Autodesk Fusion 360 part; units mm, degrees
(part 2 of 6)
sketch "b top  projection" plane through (0, 0, 0) normal (0, 0, 1) x (1, 0, 0) in component "b top component"
  arc A0 (146.8405, 15.08) -> (148.4308, 15.08) centre (147.6356, 15.6946) ccw
  arc A1 (148.4308, 24.92) -> (146.8405, 24.92) centre (147.6356, 24.3054) ccw
  arc A2 (146.825, 24.8994) -> (146.825, 23.7113) centre (147.6356, 24.3054) ccw
  arc A3 (139.8994, 3.175) -> (138.7113, 3.175) centre (139.3054, 2.3644) ccw
  arc A4 (139.92, 1.5692) -> (139.92, 3.1595) centre (139.3054, 2.3644) ccw
  arc A5 (146.825, 36.2887) -> (146.825, 35.1006) centre (147.6356, 35.6946) ccw
  arc A6 (146.8405, 35.08) -> (148.4308, 35.08) centre (147.6356, 35.6946) ccw
  arc A7 (130.08, 3.1595) -> (130.08, 1.5692) centre (130.6946, 2.3644) ccw
  arc A8 (131.2887, 3.175) -> (130.1006, 3.175) centre (130.6946, 2.3644) ccw
  arc A9 (148.4308, 44.92) -> (146.8405, 44.92) centre (147.6356, 44.3054) ccw
  arc A10 (146.825, 44.8994) -> (146.825, 43.7113) centre (147.6356, 44.3054) ccw
  arc A11 (119.8994, 3.175) -> (118.7113, 3.175) centre (119.3054, 2.3644) ccw
  arc A12 (119.92, 1.5692) -> (119.92, 3.1595) centre (119.3054, 2.3644) ccw
  arc A13 (146.825, 56.2887) -> (146.825, 55.1006) centre (147.6356, 55.6946) ccw
  arc A14 (146.8405, 55.08) -> (148.4308, 55.08) centre (147.6356, 55.6946) ccw
  arc A15 (110.08, 3.1595) -> (110.08, 1.5692) centre (110.6946, 2.3644) ccw
  arc A16 (111.2887, 3.175) -> (110.1006, 3.175) centre (110.6946, 2.3644) ccw
  arc A17 (148.4308, 64.92) -> (146.8405, 64.92) centre (147.6356, 64.3054) ccw
  arc A18 (146.825, 64.8994) -> (146.825, 63.7113) centre (147.6356, 64.3054) ccw
  arc A19 (99.8994, 3.175) -> (98.7113, 3.175) centre (99.3054, 2.3644) ccw
  arc A20 (99.92, 1.5692) -> (99.92, 3.1595) centre (99.3054, 2.3644) ccw
  arc A21 (146.825, 76.2887) -> (146.825, 75.1006) centre (147.6356, 75.6946) ccw
  arc A22 (146.8405, 75.08) -> (148.4308, 75.08) centre (147.6356, 75.6946) ccw
  arc A23 (90.08, 3.1595) -> (90.08, 1.5692) centre (90.6946, 2.3644) ccw
  arc A24 (91.2887, 3.175) -> (90.1006, 3.175) centre (90.6946, 2.3644) ccw
  arc A25 (148.4308, 84.92) -> (146.8405, 84.92) centre (147.6356, 84.3054) ccw
  arc A26 (146.825, 84.8994) -> (146.825, 83.7113) centre (147.6356, 84.3054) ccw
  arc A27 (79.8994, 3.175) -> (78.7113, 3.175) centre (79.3054, 2.3644) ccw
  arc A28 (79.92, 1.5692) -> (79.92, 3.1595) centre (79.3054, 2.3644) ccw
  arc A29 (70.08, 3.1595) -> (70.08, 1.5692) centre (70.6946, 2.3644) ccw
  arc A30 (71.2887, 3.175) -> (70.1006, 3.175) centre (70.6946, 2.3644) ccw
  arc A31 (146.825, 96.2887) -> (146.825, 95.1006) centre (147.6356, 95.6946) ccw
  arc A32 (146.8405, 95.08) -> (148.4308, 95.08) centre (147.6356, 95.6946) ccw
  arc A33 (148.4308, 104.92) -> (146.8405, 104.92) centre (147.6356, 104.3054) ccw
  arc A34 (146.825, 104.8994) -> (146.825, 103.7113) centre (147.6356, 104.3054) ccw
  arc A35 (59.8994, 3.175) -> (58.7113, 3.175) centre (59.3054, 2.3644) ccw
  arc A36 (59.92, 1.5692) -> (59.92, 3.1595) centre (59.3054, 2.3644) ccw
  arc A37 (50.08, 3.1595) -> (50.08, 1.5692) centre (50.6946, 2.3644) ccw
  arc A38 (51.2887, 3.175) -> (50.1006, 3.175) centre (50.6946, 2.3644) ccw
  arc A39 (138.7113, 116.825) -> (139.8994, 116.825) centre (139.3054, 117.6356) ccw
  arc A40 (139.92, 116.8405) -> (139.92, 118.4308) centre (139.3054, 117.6356) ccw
  arc A41 (39.8994, 3.175) -> (38.7113, 3.175) centre (39.3054, 2.3644) ccw
  arc A42 (39.92, 1.5692) -> (39.92, 3.1595) centre (39.3054, 2.3644) ccw
  arc A43 (130.08, 118.4308) -> (130.08, 116.8405) centre (130.6946, 117.6356) ccw
  arc A44 (130.1006, 116.825) -> (131.2887, 116.825) centre (130.6946, 117.6356) ccw
  arc A45 (30.08, 3.1595) -> (30.08, 1.5692) centre (30.6946, 2.3644) ccw
  arc A46 (31.2887, 3.175) -> (30.1006, 3.175) centre (30.6946, 2.3644) ccw
  arc A47 (118.7113, 116.825) -> (119.8994, 116.825) centre (119.3054, 117.6356) ccw
  arc A48 (119.92, 116.8405) -> (119.92, 118.4308) centre (119.3054, 117.6356) ccw
  arc A49 (19.8994, 3.175) -> (18.7113, 3.175) centre (19.3054, 2.3644) ccw
  arc A50 (19.92, 1.5692) -> (19.92, 3.1595) centre (19.3054, 2.3644) ccw
  arc A51 (110.08, 118.4308) -> (110.08, 116.8405) centre (110.6946, 117.6356) ccw
  arc A52 (110.1006, 116.825) -> (111.2887, 116.825) centre (110.6946, 117.6356) ccw
  arc A53 (10.08, 3.1595) -> (10.08, 1.5692) centre (10.6946, 2.3644) ccw
  arc A54 (11.2887, 3.175) -> (10.1006, 3.175) centre (10.6946, 2.3644) ccw
  arc A55 (98.7113, 116.825) -> (99.8994, 116.825) centre (99.3054, 117.6356) ccw
  arc A56 (99.92, 116.8405) -> (99.92, 118.4308) centre (99.3054, 117.6356) ccw
  arc A57 (90.08, 118.4308) -> (90.08, 116.8405) centre (90.6946, 117.6356) ccw
  arc A58 (90.1006, 116.825) -> (91.2887, 116.825) centre (90.6946, 117.6356) ccw
  arc A59 (3.175, 15.1006) -> (3.175, 16.2887) centre (2.3644, 15.6946) ccw
  arc A60 (1.5692, 15.08) -> (3.1595, 15.08) centre (2.3644, 15.6946) ccw
  arc A61 (3.1595, 24.92) -> (1.5692, 24.92) centre (2.3644, 24.3054) ccw
  arc A62 (3.175, 23.7113) -> (3.175, 24.8994) centre (2.3644, 24.3054) ccw
  arc A63 (78.7113, 116.825) -> (79.8994, 116.825) centre (79.3054, 117.6356) ccw
  arc A64 (79.92, 116.8405) -> (79.92, 118.4308) centre (79.3054, 117.6356) ccw
  arc A65 (3.175, 35.1006) -> (3.175, 36.2887) centre (2.3644, 35.6946) ccw
  arc A66 (1.5692, 35.08) -> (3.1595, 35.08) centre (2.3644, 35.6946) ccw
  arc A67 (70.08, 118.4308) -> (70.08, 116.8405) centre (70.6946, 117.6356) ccw
  arc A68 (70.1006, 116.825) -> (71.2887, 116.825) centre (70.6946, 117.6356) ccw
  arc A69 (3.1595, 44.92) -> (1.5692, 44.92) centre (2.3644, 44.3054) ccw
  arc A70 (3.175, 43.7113) -> (3.175, 44.8994) centre (2.3644, 44.3054) ccw
  arc A71 (58.7113, 116.825) -> (59.8994, 116.825) centre (59.3054, 117.6356) ccw
  arc A72 (59.92, 116.8405) -> (59.92, 118.4308) centre (59.3054, 117.6356) ccw
  arc A73 (3.175, 55.1006) -> (3.175, 56.2887) centre (2.3644, 55.6946) ccw
  arc A74 (1.5692, 55.08) -> (3.1595, 55.08) centre (2.3644, 55.6946) ccw
  arc A75 (50.08, 118.4308) -> (50.08, 116.8405) centre (50.6946, 117.6356) ccw
  arc A76 (50.1006, 116.825) -> (51.2887, 116.825) centre (50.6946, 117.6356) ccw
  arc A77 (3.1595, 64.92) -> (1.5692, 64.92) centre (2.3644, 64.3054) ccw
  arc A78 (3.175, 63.7113) -> (3.175, 64.8994) centre (2.3644, 64.3054) ccw
  arc A79 (38.7113, 116.825) -> (39.8994, 116.825) centre (39.3054, 117.6356) ccw
  arc A80 (39.92, 116.8405) -> (39.92, 118.4308) centre (39.3054, 117.6356) ccw
  arc A81 (3.175, 75.1006) -> (3.175, 76.2887) centre (2.3644, 75.6946) ccw
  arc A82 (1.5692, 75.08) -> (3.1595, 75.08) centre (2.3644, 75.6946) ccw
  arc A83 (30.08, 118.4308) -> (30.08, 116.8405) centre (30.6946, 117.6356) ccw
  arc A84 (30.1006, 116.825) -> (31.2887, 116.825) centre (30.6946, 117.6356) ccw
  arc A85 (3.1595, 84.92) -> (1.5692, 84.92) centre (2.3644, 84.3054) ccw
  arc A86 (3.175, 83.7113) -> (3.175, 84.8994) centre (2.3644, 84.3054) ccw
  arc A87 (18.7113, 116.825) -> (19.8994, 116.825) centre (19.3054, 117.6356) ccw
  arc A88 (19.92, 116.8405) -> (19.92, 118.4308) centre (19.3054, 117.6356) ccw
  arc A89 (3.175, 95.1006) -> (3.175, 96.2887) centre (2.3644, 95.6946) ccw
  arc A90 (1.5692, 95.08) -> (3.1595, 95.08) centre (2.3644, 95.6946) ccw
  arc A91 (10.08, 118.4308) -> (10.08, 116.8405) centre (10.6946, 117.6356) ccw
  arc A92 (10.1006, 116.825) -> (11.2887, 116.825) centre (10.6946, 117.6356) ccw
  arc A93 (3.1595, 104.92) -> (1.5692, 104.92) centre (2.3644, 104.3054) ccw
  arc A94 (3.175, 103.7113) -> (3.175, 104.8994) centre (2.3644, 104.3054) ccw
  arc A95 (146.825, 16.2887) -> (146.825, 15.1006) centre (147.6356, 15.6946) ccw
  line L0 (150, 15.08) -> (148.4308, 15.08)
  line L1 (146.825, 24.8994) -> (146.825, 24.92)
  line L2 (146.825, 16.2887) -> (146.825, 23.7113)
  line L3 (146.825, 15.08) -> (146.825, 15.1006)
  line L4 (148.4308, 24.92) -> (150, 24.92)
  line L5 (139.92, 3.175) -> (139.92, 3.1595)
  line L6 (146.8405, 35.08) -> (146.825, 35.08)
  line L7 (130.08, 3.175) -> (130.1006, 3.175)
  line L8 (131.2887, 3.175) -> (138.7113, 3.175)
  line L9 (130.08, 0) -> (130.08, 1.5692)
  line L10 (146.825, 44.8994) -> (146.825, 44.92)
  line L11 (146.825, 36.2887) -> (146.825, 43.7113)
  line L12 (148.4308, 44.92) -> (150, 44.92)
  line L13 (119.92, 3.175) -> (119.92, 3.1595)
  line L14 (146.8405, 55.08) -> (146.825, 55.08)
  line L15 (110.08, 3.175) -> (110.1006, 3.175)
  line L16 (111.2887, 3.175) -> (118.7113, 3.175)
  line L17 (110.08, 0) -> (110.08, 1.5692)
  line L18 (146.825, 64.8994) -> (146.825, 64.92)
  line L19 (146.825, 56.2887) -> (146.825, 63.7113)
  line L20 (99.92, 3.175) -> (99.92, 3.1595)
  line L21 (148.4308, 64.92) -> (150, 64.92)
  line L22 (146.8405, 75.08) -> (146.825, 75.08)
  line L23 (90.08, 3.175) -> (90.1006, 3.175)
  line L24 (91.2887, 3.175) -> (98.7113, 3.175)
  line L25 (90.08, 0) -> (90.08, 1.5692)
  line L26 (146.825, 84.8994) -> (146.825, 84.92)
  line L27 (146.825, 76.2887) -> (146.825, 83.7113)
  line L28 (79.92, 3.175) -> (79.92, 3.1595)
  line L29 (148.4308, 84.92) -> (150, 84.92)
  line L30 (70.08, 3.175) -> (70.1006, 3.175)
  line L31 (71.2887, 3.175) -> (78.7113, 3.175)
  line L32 (146.8405, 95.08) -> (146.825, 95.08)
  line L33 (70.08, 0) -> (70.08, 1.5692)
  line L34 (146.825, 104.8994) -> (146.825, 104.92)
  line L35 (146.825, 96.2887) -> (146.825, 103.7113)
  line L36 (59.92, 3.175) -> (59.92, 3.1595)
  line L37 (148.4308, 104.92) -> (150, 104.92)
  line L38 (50.08, 3.175) -> (50.1006, 3.175)
  line L39 (51.2887, 3.175) -> (58.7113, 3.175)
  line L40 (139.92, 116.825) -> (139.92, 116.8405)
  line L41 (50.08, 0) -> (50.08, 1.5692)
  line L42 (130.08, 116.825) -> (130.1006, 116.825)
  line L43 (131.2887, 116.825) -> (138.7113, 116.825)
  line L44 (39.92, 3.175) -> (39.92, 3.1595)
  line L45 (130.08, 120) -> (130.08, 118.4308)
  line L46 (30.08, 3.175) -> (30.1006, 3.175)
  line L47 (31.2887, 3.175) -> (38.7113, 3.175)
  line L48 (119.92, 116.825) -> (119.92, 116.8405)
  line L49 (30.08, 0) -> (30.08, 1.5692)
  line L50 (110.08, 116.825) -> (110.1006, 116.825)
  line L51 (111.2887, 116.825) -> (118.7113, 116.825)
  line L52 (19.92, 3.175) -> (19.92, 3.1595)
  line L53 (110.08, 120) -> (110.08, 118.4308)
  line L54 (10.08, 3.175) -> (10.1006, 3.175)
  line L55 (11.2887, 3.175) -> (18.7113, 3.175)
  line L56 (99.92, 116.825) -> (99.92, 116.8405)
  line L57 (10.08, 0) -> (10.08, 1.5692)
  line L58 (90.08, 116.825) -> (90.1006, 116.825)
  line L59 (91.2887, 116.825) -> (98.7113, 116.825)
  line L60 (3.1595, 15.08) -> (3.175, 15.08)
  line L61 (90.08, 120) -> (90.08, 118.4308)
  line L62 (3.175, 24.8994) -> (3.175, 24.92)
  line L63 (3.175, 16.2887) -> (3.175, 23.7113)
  line L64 (79.92, 116.825) -> (79.92, 116.8405)
  line L65 (1.5692, 24.92) -> (0, 24.92)
  line L66 (70.08, 116.825) -> (70.1006, 116.825)
  line L67 (71.2887, 116.825) -> (78.7113, 116.825)
  line L68 (3.1595, 35.08) -> (3.175, 35.08)
  line L69 (70.08, 120) -> (70.08, 118.4308)
  line L70 (3.175, 44.8994) -> (3.175, 44.92)
  line L71 (3.175, 36.2887) -> (3.175, 43.7113)
  line L72 (59.92, 116.825) -> (59.92, 116.8405)
  line L73 (1.5692, 44.92) -> (0, 44.92)
  line L74 (3.1595, 55.08) -> (3.175, 55.08)
  line L75 (50.08, 116.825) -> (50.1006, 116.825)
  line L76 (51.2887, 116.825) -> (58.7113, 116.825)
  line L77 (50.08, 120) -> (50.08, 118.4308)
  line L78 (3.175, 64.8994) -> (3.175, 64.92)
  line L79 (3.175, 56.2887) -> (3.175, 63.7113)
  line L80 (1.5692, 64.92) -> (0, 64.92)
  line L81 (39.92, 116.825) -> (39.92, 116.8405)
  line L82 (3.1595, 75.08) -> (3.175, 75.08)
  line L83 (30.08, 116.825) -> (30.1006, 116.825)
  line L84 (31.2887, 116.825) -> (38.7113, 116.825)
  line L85 (3.175, 84.8994) -> (3.175, 84.92)
  line L86 (3.175, 76.2887) -> (3.175, 83.7113)
  line L87 (30.08, 120) -> (30.08, 118.4308)
  line L88 (1.5692, 84.92) -> (0, 84.92)
  line L89 (19.92, 116.825) -> (19.92, 116.8405)
  line L90 (3.1595, 95.08) -> (3.175, 95.08)
  line L91 (10.08, 116.825) -> (10.1006, 116.825)
  line L92 (11.2887, 116.825) -> (18.7113, 116.825)
  line L93 (3.175, 104.8994) -> (3.175, 104.92)
  line L94 (3.175, 96.2887) -> (3.175, 103.7113)
  line L95 (10.08, 120) -> (10.08, 118.4308)
  line L96 (1.5692, 104.92) -> (0, 104.92)
  line L97 (0, 0) -> (0, 15.08)
  line L98 (0, 15.08) -> (1.5692, 15.08)
  line L99 (3.175, 15.08) -> (3.175, 15.1006)
  line L100 (3.175, 24.92) -> (3.1595, 24.92)
  line L101 (0, 24.92) -> (0, 35.08)
  line L102 (0, 35.08) -> (1.5692, 35.08)
  line L103 (3.175, 35.08) -> (3.175, 35.1006)
  line L104 (3.175, 44.92) -> (3.1595, 44.92)
  line L105 (0, 44.92) -> (0, 55.08)
  line L106 (0, 55.08) -> (1.5692, 55.08)
  line L107 (3.175, 55.08) -> (3.175, 55.1006)
  line L108 (3.175, 64.92) -> (3.1595, 64.92)
  line L109 (0, 64.92) -> (0, 75.08)
  line L110 (0, 75.08) -> (1.5692, 75.08)
  line L111 (3.175, 75.08) -> (3.175, 75.1006)
  line L112 (3.175, 84.92) -> (3.1595, 84.92)
  line L113 (0, 84.92) -> (0, 95.08)
  line L114 (0, 95.08) -> (1.5692, 95.08)
  line L115 (3.175, 95.08) -> (3.175, 95.1006)
  line L116 (3.175, 104.92) -> (3.1595, 104.92)
  line L117 (0, 104.92) -> (0, 120)
  line L118 (0, 120) -> (10.08, 120)
  line L119 (10.08, 116.8405) -> (10.08, 116.825)
  line L120 (19.8994, 116.825) -> (19.92, 116.825)
  line L121 (19.92, 118.4308) -> (19.92, 120)
  line L122 (19.92, 120) -> (30.08, 120)
  line L123 (30.08, 116.8405) -> (30.08, 116.825)
  line L124 (39.8994, 116.825) -> (39.92, 116.825)
  line L125 (39.92, 118.4308) -> (39.92, 120)
  line L126 (39.92, 120) -> (50.08, 120)
  line L127 (50.08, 116.8405) -> (50.08, 116.825)
  line L128 (59.8994, 116.825) -> (59.92, 116.825)
  line L129 (59.92, 118.4308) -> (59.92, 120)
  line L130 (59.92, 120) -> (70.08, 120)
  line L131 (70.08, 116.8405) -> (70.08, 116.825)
  line L132 (79.8994, 116.825) -> (79.92, 116.825)
  line L133 (79.92, 118.4308) -> (79.92, 120)
  line L134 (79.92, 120) -> (90.08, 120)
  line L135 (90.08, 116.8405) -> (90.08, 116.825)
  line L136 (99.8994, 116.825) -> (99.92, 116.825)
  line L137 (99.92, 118.4308) -> (99.92, 120)
  line L138 (99.92, 120) -> (110.08, 120)
  line L139 (110.08, 116.8405) -> (110.08, 116.825)
  line L140 (119.8994, 116.825) -> (119.92, 116.825)
  line L141 (119.92, 118.4308) -> (119.92, 120)
  line L142 (119.92, 120) -> (130.08, 120)
  line L143 (130.08, 116.8405) -> (130.08, 116.825)
  line L144 (139.8994, 116.825) -> (139.92, 116.825)
  line L145 (139.92, 118.4308) -> (139.92, 120)
  line L146 (139.92, 120) -> (150, 120)
  line L147 (150, 104.92) -> (150, 120)
  line L148 (146.825, 104.92) -> (146.8405, 104.92)
  line L149 (146.825, 95.08) -> (146.825, 95.1006)
  line L150 (150, 95.08) -> (148.4308, 95.08)
  line L151 (150, 84.92) -> (150, 95.08)
  line L152 (146.825, 84.92) -> (146.8405, 84.92)
  line L153 (146.825, 75.08) -> (146.825, 75.1006)
  line L154 (150, 75.08) -> (148.4308, 75.08)
  line L155 (150, 64.92) -> (150, 75.08)
  line L156 (146.825, 64.92) -> (146.8405, 64.92)
  line L157 (146.825, 55.08) -> (146.825, 55.1006)
  line L158 (150, 55.08) -> (148.4308, 55.08)
  line L159 (150, 44.92) -> (150, 55.08)
  line L160 (146.825, 44.92) -> (146.8405, 44.92)
  line L161 (146.825, 35.08) -> (146.825, 35.1006)
  line L162 (150, 35.08) -> (148.4308, 35.08)
  line L163 (150, 24.92) -> (150, 35.08)
  line L164 (146.825, 24.92) -> (146.8405, 24.92)
  line L165 (146.8405, 15.08) -> (146.825, 15.08)
  line L166 (150, 0) -> (150, 15.08)
  line L167 (139.92, 0) -> (150, 0)
  line L168 (139.92, 1.5692) -> (139.92, 0)
  line L169 (139.8994, 3.175) -> (139.92, 3.175)
  line L170 (130.08, 3.1595) -> (130.08, 3.175)
  line L171 (119.92, 0) -> (130.08, 0)
  line L172 (119.92, 1.5692) -> (119.92, 0)
  line L173 (119.8994, 3.175) -> (119.92, 3.175)
  line L174 (110.08, 3.1595) -> (110.08, 3.175)
  line L175 (99.92, 0) -> (110.08, 0)
  line L176 (99.92, 1.5692) -> (99.92, 0)
  line L177 (99.8994, 3.175) -> (99.92, 3.175)
  line L178 (90.08, 3.1595) -> (90.08, 3.175)
  line L179 (79.92, 0) -> (90.08, 0)
  line L180 (79.92, 1.5692) -> (79.92, 0)
  line L181 (79.8994, 3.175) -> (79.92, 3.175)
  line L182 (70.08, 3.1595) -> (70.08, 3.175)
  line L183 (59.92, 0) -> (70.08, 0)
  line L184 (59.92, 1.5692) -> (59.92, 0)
  line L185 (59.8994, 3.175) -> (59.92, 3.175)
  line L186 (50.08, 3.1595) -> (50.08, 3.175)
  line L187 (39.92, 0) -> (50.08, 0)
  line L188 (39.92, 1.5692) -> (39.92, 0)
  line L189 (39.8994, 3.175) -> (39.92, 3.175)
  line L190 (30.08, 3.1595) -> (30.08, 3.175)
  line L191 (19.92, 0) -> (30.08, 0)
  line L192 (19.92, 1.5692) -> (19.92, 0)
  line L193 (19.8994, 3.175) -> (19.92, 3.175)
  line L194 (10.08, 3.1595) -> (10.08, 3.175)
  line L195 (0, 0) -> (10.08, 0)
sketch "b bottom lines" plane through (0, 0, 0) normal (0, 0, 1) x (1, 0, 0) in component "b bottom component"
  line L0 (152.01, 0) -> (162.09, 0)
  line L1 (162.09, 0) -> (162.09, 3.175)
  line L2 (162.09, 3.175) -> (171.93, 3.175)
  line L3 (171.93, 3.175) -> (171.93, 0)
  line L4 (171.93, 0) -> (182.09, 0)
  line L5 (182.09, 0) -> (182.09, 3.175)
  line L6 (182.09, 3.175) -> (191.93, 3.175)
  line L7 (191.93, 3.175) -> (191.93, 0)
  line L8 (191.93, 0) -> (202.09, 0)
  line L9 (202.09, 0) -> (202.09, 3.175)
  line L10 (202.09, 3.175) -> (211.93, 3.175)
  line L11 (211.93, 3.175) -> (211.93, 0)
  line L12 (211.93, 0) -> (222.09, 0)
  line L13 (222.09, 0) -> (222.09, 3.175)
  line L14 (222.09, 3.175) -> (231.93, 3.175)
  line L15 (231.93, 3.175) -> (231.93, 0)
  line L16 (231.93, 0) -> (242.09, 0)
  line L17 (242.09, 0) -> (242.09, 3.175)
  line L18 (242.09, 3.175) -> (251.93, 3.175)
  line L19 (251.93, 3.175) -> (251.93, 0)
  line L20 (251.93, 0) -> (262.09, 0)
  line L21 (262.09, 0) -> (262.09, 3.175)
  line L22 (262.09, 3.175) -> (271.93, 3.175)
  line L23 (271.93, 3.175) -> (271.93, 0)
  line L24 (271.93, 0) -> (282.09, 0)
  line L25 (282.09, 0) -> (282.09, 3.175)
  line L26 (282.09, 3.175) -> (291.93, 3.175)
  line L27 (291.93, 3.175) -> (291.93, 0)
  line L28 (291.93, 0) -> (302.01, 0)
  line L29 (302.01, 0) -> (302.01, 15.08)
  line L30 (302.01, 15.08) -> (298.835, 15.08)
  line L31 (298.835, 15.08) -> (298.835, 24.92)
  line L32 (298.835, 24.92) -> (302.01, 24.92)
  line L33 (302.01, 24.92) -> (302.01, 35.08)
  line L34 (302.01, 35.08) -> (298.835, 35.08)
  line L35 (298.835, 35.08) -> (298.835, 44.92)
  line L36 (298.835, 44.92) -> (302.01, 44.92)
  line L37 (302.01, 44.92) -> (302.01, 55.08)
  line L38 (302.01, 55.08) -> (298.835, 55.08)
  line L39 (298.835, 55.08) -> (298.835, 64.92)
  line L40 (298.835, 64.92) -> (302.01, 64.92)
  line L41 (302.01, 64.92) -> (302.01, 75.08)
  line L42 (302.01, 75.08) -> (298.835, 75.08)
  line L43 (298.835, 75.08) -> (298.835, 84.92)
  line L44 (298.835, 84.92) -> (302.01, 84.92)
  line L45 (302.01, 84.92) -> (302.01, 95.08)
  line L46 (302.01, 95.08) -> (298.835, 95.08)
  line L47 (298.835, 95.08) -> (298.835, 104.92)
  line L48 (298.835, 104.92) -> (302.01, 104.92)
  line L49 (302.01, 104.92) -> (302.01, 120)
  line L50 (152.01, 120) -> (162.09, 120)
  line L51 (162.09, 120) -> (162.09, 116.825)
  line L52 (162.09, 116.825) -> (171.93, 116.825)
  line L53 (171.93, 116.825) -> (171.93, 120)
  line L54 (171.93, 120) -> (182.09, 120)
  line L55 (182.09, 120) -> (182.09, 116.825)
  line L56 (182.09, 116.825) -> (191.93, 116.825)
  line L57 (191.93, 116.825) -> (191.93, 120)
  line L58 (191.93, 120) -> (202.09, 120)
  line L59 (202.09, 120) -> (202.09, 116.825)
  line L60 (202.09, 116.825) -> (211.93, 116.825)
  line L61 (211.93, 116.825) -> (211.93, 120)
  line L62 (211.93, 120) -> (222.09, 120)
  line L63 (222.09, 120) -> (222.09, 116.825)
  line L64 (222.09, 116.825) -> (231.93, 116.825)
  line L65 (231.93, 116.825) -> (231.93, 120)
  line L66 (231.93, 120) -> (242.09, 120)
  line L67 (242.09, 120) -> (242.09, 116.825)
  line L68 (242.09, 116.825) -> (251.93, 116.825)
  line L69 (251.93, 116.825) -> (251.93, 120)
  line L70 (251.93, 120) -> (262.09, 120)
  line L71 (262.09, 120) -> (262.09, 116.825)
  line L72 (262.09, 116.825) -> (271.93, 116.825)
  line L73 (271.93, 116.825) -> (271.93, 120)
  line L74 (271.93, 120) -> (282.09, 120)
  line L75 (282.09, 120) -> (282.09, 116.825)
  line L76 (282.09, 116.825) -> (291.93, 116.825)
  line L77 (291.93, 116.825) -> (291.93, 120)
  line L78 (291.93, 120) -> (302.01, 120)
  line L79 (152.01, 0) -> (152.01, 15.08)
  line L80 (152.01, 15.08) -> (155.185, 15.08)
  line L81 (155.185, 15.08) -> (155.185, 24.92)
  line L82 (155.185, 24.92) -> (152.01, 24.92)
  line L83 (152.01, 24.92) -> (152.01, 35.08)
  line L84 (152.01, 35.08) -> (155.185, 35.08)
  line L85 (155.185, 35.08) -> (155.185, 44.92)
  line L86 (155.185, 44.92) -> (152.01, 44.92)
  line L87 (152.01, 44.92) -> (152.01, 55.08)
  line L88 (152.01, 55.08) -> (155.185, 55.08)
  line L89 (155.185, 55.08) -> (155.185, 64.92)
  line L90 (155.185, 64.92) -> (152.01, 64.92)
  line L91 (152.01, 64.92) -> (152.01, 75.08)
  line L92 (152.01, 75.08) -> (155.185, 75.08)
  line L93 (155.185, 75.08) -> (155.185, 84.92)
  line L94 (155.185, 84.92) -> (152.01, 84.92)
  line L95 (152.01, 84.92) -> (152.01, 95.08)
  line L96 (152.01, 95.08) -> (155.185, 95.08)
  line L97 (155.185, 95.08) -> (155.185, 104.92)
  line L98 (155.185, 104.92) -> (152.01, 104.92)
  line L99 (152.01, 104.92) -> (152.01, 120)
  dimension "d5342" = 10.08
  dimension "d5343" = 3.175
  dimension "d5344" = 9.84
  dimension "d5345" = 3.175
  dimension "d5346" = 10.16
  dimension "d5347" = 3.175
  dimension "d5348" = 9.84
  dimension "d5349" = 3.175
  dimension "d5350" = 10.16
  dimension "d5351" = 3.175
  dimension "d5352" = 9.84
  dimension "d5353" = 3.175
  dimension "d5354" = 10.16
  dimension "d5355" = 3.175
  dimension "d5356" = 9.84
  dimension "d5357" = 3.175
  dimension "d5358" = 10.16
  dimension "d5359" = 3.175
  dimension "d5360" = 9.84
  dimension "d5361" = 3.175
  dimension "d5362" = 10.16
  dimension "d5363" = 3.175
  dimension "d5364" = 9.84
  dimension "d5365" = 3.175
  dimension "d5366" = 10.16
  dimension "d5367" = 3.175
  dimension "d5368" = 9.84
  dimension "d5369" = 3.175
  dimension "d5370" = 10.08
  dimension "d5385" = 15.08
  dimension "d5386" = 3.175
  dimension "d5387" = 9.84
  dimension "d5388" = 3.175
  dimension "d5389" = 10.16
  dimension "d5390" = 3.175
  dimension "d5391" = 9.84
  dimension "d5392" = 3.175
  dimension "d5393" = 10.16
  dimension "d5394" = 3.175
  dimension "d5395" = 9.84
  dimension "d5396" = 3.175
  dimension "d5397" = 10.16
  dimension "d5398" = 3.175
  dimension "d5399" = 9.84
  dimension "d5400" = 3.175
  dimension "d5401" = 10.16
  dimension "d5402" = 3.175
  dimension "d5403" = 9.84
  dimension "d5404" = 3.175
  dimension "d5405" = 15.08
  dimension "d5416" = 10.08
  dimension "d5417" = 3.175
  dimension "d5418" = 9.84
  dimension "d5419" = 3.175
  dimension "d5420" = 10.16
  dimension "d5421" = 3.175
  dimension "d5422" = 9.84
  dimension "d5423" = 3.175
  dimension "d5424" = 10.16
  dimension "d5425" = 3.175
  dimension "d5426" = 9.84
  dimension "d5427" = 3.175
  dimension "d5428" = 10.16
  dimension "d5429" = 3.175
  dimension "d5430" = 9.84
  dimension "d5431" = 3.175
  dimension "d5432" = 10.16
  dimension "d5433" = 3.175
  dimension "d5434" = 9.84
  dimension "d5435" = 3.175
  dimension "d5436" = 10.16
  dimension "d5437" = 3.175
  dimension "d5438" = 9.84
  dimension "d5439" = 3.175
  dimension "d5440" = 10.16
  dimension "d5441" = 3.175
  dimension "d5442" = 9.84
  dimension "d5443" = 3.175
  dimension "d5444" = 10.08
  dimension "d5459" = 15.08
  dimension "d5460" = 3.175
  dimension "d5461" = 9.84
  dimension "d5462" = 3.175
  dimension "d5463" = 10.16
  dimension "d5464" = 3.175
  dimension "d5465" = 9.84
  dimension "d5466" = 3.175
  dimension "d5467" = 10.16
  dimension "d5468" = 3.175
  dimension "d5469" = 9.84
  dimension "d5470" = 3.175
  dimension "d5471" = 10.16
  dimension "d5472" = 3.175
  dimension "d5473" = 9.84
  dimension "d5474" = 3.175
  dimension "d5475" = 10.16
  dimension "d5476" = 3.175
  dimension "d5477" = 9.84
  dimension "d5478" = 3.175
  dimension "d5479" = 15.08
  constraint horizontal L0
  constraint vertical L1
  constraint horizontal L2
  constraint vertical L3
  constraint horizontal L4
  constraint vertical L5
  constraint horizontal L6
  constraint vertical L7
  constraint horizontal L8
  constraint vertical L9
  constraint horizontal L10
  constraint vertical L11
  constraint horizontal L12
  constraint vertical L13
  constraint horizontal L14
  constraint vertical L15
  constraint horizontal L16
  constraint vertical L17
  constraint horizontal L18
  constraint vertical L19
  constraint horizontal L20
  constraint vertical L21
  constraint horizontal L22
  constraint vertical L23
  constraint horizontal L24
  constraint vertical L25
  constraint horizontal L26
  constraint vertical L27
  constraint horizontal L28
  constraint vertical L29
  constraint horizontal L30
  constraint vertical L31
  constraint horizontal L32
  constraint vertical L33
  constraint horizontal L34
  constraint vertical L35
  constraint horizontal L36
  constraint vertical L37
  constraint horizontal L38
  constraint vertical L39
  constraint horizontal L40
  constraint vertical L41
  constraint horizontal L42
  constraint vertical L43
  constraint horizontal L44
  constraint vertical L45
  constraint horizontal L46
  constraint vertical L47
  constraint horizontal L48
  constraint vertical L49
  constraint horizontal L50
  constraint vertical L51
  constraint horizontal L52
  constraint vertical L53
  constraint horizontal L54
  constraint vertical L55
  constraint horizontal L56
  constraint vertical L57
  constraint horizontal L58
  constraint vertical L59
  constraint horizontal L60
  constraint vertical L61
  constraint horizontal L62
  constraint vertical L63
  constraint horizontal L64
  constraint vertical L65
  constraint horizontal L66
  constraint vertical L67
  constraint horizontal L68
  constraint vertical L69
  constraint horizontal L70
  constraint vertical L71
  constraint horizontal L72
  constraint vertical L73
  constraint horizontal L74
  constraint vertical L75
  constraint horizontal L76
  constraint vertical L77
  constraint horizontal L78
  constraint vertical L79
  constraint horizontal L80
  constraint vertical L81
  constraint horizontal L82
  constraint vertical L83
  constraint horizontal L84
  constraint vertical L85
  constraint horizontal L86
  constraint vertical L87
  constraint horizontal L88
  constraint vertical L89
  constraint horizontal L90
  constraint vertical L91
  constraint horizontal L92
  constraint vertical L93
  constraint horizontal L94
  constraint vertical L95
  constraint horizontal L96
  constraint vertical L97
  constraint horizontal L98
  constraint vertical L99
  measures "d5342" distance of L0.start L0.end
  measures "d5343" distance of L0.end L1.end
  measures "d5344" distance of L1.end L2.end
  measures "d5345" distance of L2.end L3.end
  measures "d5346" distance of L3.end L4.end
  measures "d5347" distance of L4.end L5.end
  measures "d5348" distance of L5.end L6.end
  measures "d5349" distance of L6.end L7.end
  measures "d5350" distance of L7.end L8.end
  measures "d5351" distance of L8.end L9.end
  measures "d5352" distance of L9.end L10.end
  measures "d5353" distance of L10.end L11.end
  measures "d5354" distance of L11.end L12.end
  measures "d5355" distance of L12.end L13.end
  measures "d5356" distance of L13.end L14.end
  measures "d5357" distance of L14.end L15.end
  measures "d5358" distance of L15.end L16.end
  measures "d5359" distance of L16.end L17.end
  measures "d5360" distance of L17.end L18.end
  measures "d5361" distance of L18.end L19.end
  measures "d5362" distance of L19.end L20.end
  measures "d5363" distance of L20.end L21.end
  measures "d5364" distance of L21.end L22.end
  measures "d5365" distance of L22.end L23.end
  measures "d5366" distance of L23.end L24.end
  measures "d5367" distance of L24.end L25.end
  measures "d5368" distance of L25.end L26.end
  measures "d5369" distance of L26.end L27.end
  measures "d5370" distance of L27.end L28.end
  measures "d5385" distance of L28.end L29.end
  measures "d5386" distance of L29.end L30.end
  measures "d5387" distance of L30.end L31.end
  measures "d5388" distance of L31.end L32.end
  measures "d5389" distance of L32.end L33.end
  measures "d5390" distance of L33.end L34.end
  measures "d5391" distance of L34.end L35.end
  measures "d5392" distance of L35.end L36.end
  measures "d5393" distance of L36.end L37.end
  measures "d5394" distance of L37.end L38.end
  measures "d5395" distance of L38.end L39.end
  measures "d5396" distance of L39.end L40.end
  measures "d5397" distance of L40.end L41.end
  measures "d5398" distance of L41.end L42.end
  measures "d5399" distance of L42.end L43.end
  measures "d5400" distance of L43.end L44.end
  measures "d5401" distance of L44.end L45.end
  measures "d5402" distance of L45.end L46.end
  measures "d5403" distance of L46.end L47.end
  measures "d5404" distance of L47.end L48.end
  measures "d5405" distance of L48.end L49.end
  measures "d5416" distance of L50.start L50.end
  measures "d5417" distance of L50.end L51.end
  measures "d5418" distance of L51.end L52.end
  measures "d5419" distance of L52.end L53.end
  measures "d5420" distance of L53.end L54.end
  measures "d5421" distance of L54.end L55.end
  measures "d5422" distance of L55.end L56.end
  measures "d5423" distance of L56.end L57.end
  measures "d5424" distance of L57.end L58.end
  measures "d5425" distance of L58.end L59.end
  measures "d5426" distance of L59.end L60.end
  measures "d5427" distance of L60.end L61.end
  measures "d5428" distance of L61.end L62.end
  measures "d5429" distance of L62.end L63.end
  measures "d5430" distance of L63.end L64.end
  measures "d5431" distance of L64.end L65.end
  measures "d5432" distance of L65.end L66.end
  measures "d5433" distance of L66.end L67.end
  measures "d5434" distance of L67.end L68.end
  measures "d5435" distance of L68.end L69.end
  measures "d5436" distance of L69.end L70.end
  measures "d5437" distance of L70.end L71.end
  measures "d5438" distance of L71.end L72.end
  measures "d5439" distance of L72.end L73.end
  measures "d5440" distance of L73.end L74.end
  measures "d5441" distance of L74.end L75.end
  measures "d5442" distance of L75.end L76.end
  measures "d5443" distance of L76.end L77.end
  measures "d5444" distance of L49.end L77.end
  measures "d5459" distance of L0.start L79.end
  measures "d5460" distance of L79.end L80.end
  measures "d5461" distance of L80.end L81.end
  measures "d5462" distance of L81.end L82.end
  measures "d5463" distance of L82.end L83.end
  measures "d5464" distance of L83.end L84.end
  measures "d5465" distance of L84.end L85.end
  measures "d5466" distance of L85.end L86.end
  measures "d5467" distance of L86.end L87.end
  measures "d5468" distance of L87.end L88.end
  measures "d5469" distance of L88.end L89.end
  measures "d5470" distance of L89.end L90.end
  measures "d5471" distance of L90.end L91.end
  measures "d5472" distance of L91.end L92.end
  measures "d5473" distance of L92.end L93.end
  measures "d5474" distance of L93.end L94.end
  measures "d5475" distance of L94.end L95.end
  measures "d5476" distance of L95.end L96.end
  measures "d5477" distance of L96.end L97.end
  measures "d5478" distance of L97.end L98.end
  measures "d5479" distance of L50.start L98.end
sketch "b bottom circles" plane through (0, 0, 0) normal (0, 0, 1) x (1, 0, 0) in component "b bottom component"
  line L0 (152.01, 0) -> (302.01, 0)
  line L1 (302.01, 0) -> (302.01, 120)
  line L2 (302.01, 120) -> (152.01, 120)
  line L3 (152.01, 120) -> (152.01, 0)
  circle A0 centre (162.7046, 2.3644) radius 1.005
  circle A1 centre (171.3154, 2.3644) radius 1.005
  circle A2 centre (182.7046, 2.3644) radius 1.005
  circle A3 centre (191.3154, 2.3644) radius 1.005
  circle A4 centre (202.7046, 2.3644) radius 1.005
  circle A5 centre (211.3154, 2.3644) radius 1.005
  circle A6 centre (222.7046, 2.3644) radius 1.005
  circle A7 centre (231.3154, 2.3644) radius 1.005
  circle A8 centre (242.7046, 2.3644) radius 1.005
  circle A9 centre (251.3154, 2.3644) radius 1.005
  circle A10 centre (262.7046, 2.3644) radius 1.005
  circle A11 centre (271.3154, 2.3644) radius 1.005
  circle A12 centre (282.7046, 2.3644) radius 1.005
  circle A13 centre (291.3154, 2.3644) radius 1.005
  circle A14 centre (299.6456, 15.6946) radius 1.005
  circle A15 centre (299.6456, 24.3054) radius 1.005
  circle A16 centre (299.6456, 35.6946) radius 1.005
  circle A17 centre (299.6456, 44.3054) radius 1.005
  circle A18 centre (299.6456, 55.6946) radius 1.005
  circle A19 centre (299.6456, 64.3054) radius 1.005
  circle A20 centre (299.6456, 75.6946) radius 1.005
  circle A21 centre (299.6456, 84.3054) radius 1.005
  circle A22 centre (299.6456, 95.6946) radius 1.005
  circle A23 centre (299.6456, 104.3054) radius 1.005
  circle A24 centre (162.7046, 117.6356) radius 1.005
  circle A25 centre (171.3154, 117.6356) radius 1.005
  circle A26 centre (182.7046, 117.6356) radius 1.005
  circle A27 centre (191.3154, 117.6356) radius 1.005
  circle A28 centre (202.7046, 117.6356) radius 1.005
  circle A29 centre (211.3154, 117.6356) radius 1.005
  circle A30 centre (222.7046, 117.6356) radius 1.005
  circle A31 centre (231.3154, 117.6356) radius 1.005
  circle A32 centre (242.7046, 117.6356) radius 1.005
  circle A33 centre (251.3154, 117.6356) radius 1.005
  circle A34 centre (262.7046, 117.6356) radius 1.005
  circle A35 centre (271.3154, 117.6356) radius 1.005
  circle A36 centre (282.7046, 117.6356) radius 1.005
  circle A37 centre (291.3154, 117.6356) radius 1.005
  circle A38 centre (154.3744, 15.6946) radius 1.005
  circle A39 centre (154.3744, 24.3054) radius 1.005
  circle A40 centre (154.3744, 35.6946) radius 1.005
  circle A41 centre (154.3744, 44.3054) radius 1.005
  circle A42 centre (154.3744, 55.6946) radius 1.005
  circle A43 centre (154.3744, 64.3054) radius 1.005
  circle A44 centre (154.3744, 75.6946) radius 1.005
  circle A45 centre (154.3744, 84.3054) radius 1.005
  circle A46 centre (154.3744, 95.6946) radius 1.005
  circle A47 centre (154.3744, 104.3054) radius 1.005
  dimension "d5371" = 2.01
  dimension "d5372" = 2.01
  dimension "d5373" = 2.01
  dimension "d5374" = 2.01
  dimension "d5375" = 2.01
  dimension "d5376" = 2.01
  dimension "d5377" = 2.01
  dimension "d5378" = 2.01
  dimension "d5379" = 2.01
  dimension "d5380" = 2.01
  dimension "d5381" = 2.01
  dimension "d5382" = 2.01
  dimension "d5383" = 2.01
  dimension "d5384" = 2.01
  dimension "d5406" = 2.01
  dimension "d5407" = 2.01
  dimension "d5408" = 2.01
  dimension "d5409" = 2.01
  dimension "d5410" = 2.01
  dimension "d5411" = 2.01
  dimension "d5412" = 2.01
  dimension "d5413" = 2.01
  dimension "d5414" = 2.01
  dimension "d5415" = 2.01
  dimension "d5445" = 2.01
  dimension "d5446" = 2.01
  dimension "d5447" = 2.01
  dimension "d5448" = 2.01
  dimension "d5449" = 2.01
  dimension "d5450" = 2.01
  dimension "d5451" = 2.01
  dimension "d5452" = 2.01
  dimension "d5453" = 2.01
  dimension "d5454" = 2.01
  dimension "d5455" = 2.01
  dimension "d5456" = 2.01
  dimension "d5457" = 2.01
  dimension "d5458" = 2.01
  dimension "d5480" = 2.01
  dimension "d5481" = 2.01
  dimension "d5482" = 2.01
  dimension "d5483" = 2.01
  dimension "d5484" = 2.01
  dimension "d5485" = 2.01
  dimension "d5486" = 2.01
  dimension "d5487" = 2.01
  dimension "d5488" = 2.01
  dimension "d5489" = 2.01
  measures "d5371" diameter of A0
  measures "d5372" diameter of A1
  measures "d5373" diameter of A2
  measures "d5374" diameter of A3
  measures "d5375" diameter of A4
  measures "d5376" diameter of A5
  measures "d5377" diameter of A6
  measures "d5378" diameter of A7
  measures "d5379" diameter of A8
  measures "d5380" diameter of A9
  measures "d5381" diameter of A10
  measures "d5382" diameter of A11
  measures "d5383" diameter of A12
  measures "d5384" diameter of A13
  measures "d5406" diameter of A14
  measures "d5407" diameter of A15
  measures "d5408" diameter of A16
  measures "d5409" diameter of A17
  measures "d5410" diameter of A18
  measures "d5411" diameter of A19
  measures "d5412" diameter of A20
  measures "d5413" diameter of A21
  measures "d5414" diameter of A22
  measures "d5415" diameter of A23
  measures "d5445" diameter of A24
  measures "d5446" diameter of A25
  measures "d5447" diameter of A26
  measures "d5448" diameter of A27
  measures "d5449" diameter of A28
  measures "d5450" diameter of A29
  measures "d5451" diameter of A30
  measures "d5452" diameter of A31
  measures "d5453" diameter of A32
  measures "d5454" diameter of A33
  measures "d5455" diameter of A34
  measures "d5456" diameter of A35
  measures "d5457" diameter of A36
  measures "d5458" diameter of A37
  measures "d5480" diameter of A38
  measures "d5481" diameter of A39
  measures "d5482" diameter of A40
  measures "d5483" diameter of A41
  measures "d5484" diameter of A42
  measures "d5485" diameter of A43
  measures "d5486" diameter of A44
  measures "d5487" diameter of A45
  measures "d5488" diameter of A46
  measures "d5489" diameter of A47
extrude "b bottom lines body extrude" add sketch "b bottom lines" along normal blind 3.175 separate body makes body 4 in component "b bottom component"
extrude "b bottom circles extrude" add sketch "b bottom circles" along normal blind 3.175 separate body makes body 5 in component "b bottom component"
combine "b bottom lines final combine feature" operation intersect target body 4 tool bodies 5 in component "b bottom component"